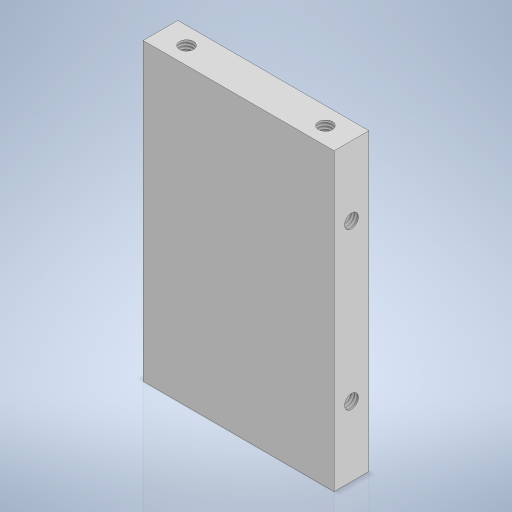
# Autodesk Inventor part: 1013
Saved by Autodesk Inventor 2024 (Build 280153000, 153)
## iProperties
Created: 2024-07-12
Part Number: 1013
Material: Generisch
Document SubType Name: Modeling
Designer: ffogue
Density: 1 g/cm^3
Appearance: Vorgabe
Author: ffogue
Autodesk Inventor part; units mm, degrees
ref_plane "XZ Plane" through (0, 0, 0) normal (0, 1, 0) x (-1, 0, 0)
sketch "Skizze1" plane through (0, 0, 0) normal (0, 1, 0) x (-1, 0, 0)
  line L0 (0, 0) -> (44, 0)
  line L1 (44, 0) -> (44, -68)
  line L2 (44, -68) -> (0, -68)
  line L3 (0, -68) -> (0, 0)
  dimension "d0" = 44
  dimension "d1" = 68
  constraints: 8 end point, 2 parallel, 1 horizontal, 1 perpendicular
  measures "d0" distance between parallel lines of L3 L1
  measures "d1" distance between parallel lines of L2 L0
extrude "Extrusion1" add sketch "Skizze1" along normal blind 8
sketch "Skizze2" plane through (-44, 0, 0) normal (0, 0, 1) x (1, 0, 0)
  line L0 (44, 0) -> (44, 8) projected
  point P0 (38, 4)
  point P1 (6, 4)
  point P2 (44, 4)
  dimension "d4" = 32
  dimension "d5" = 6
  constraints: 2 horizontal alignment, 1 midpoint
  measures "d4" distance of point (38, 4) point (6, 4)
  measures "d5" distance from line of L0 point (38, 4)
hole "Bohrung1" at (-6, 4, 0) at (-38, 4, 0) direction (0, 0, -1) diameter 3.242 depth 10 thread size "M4x0.7" class "6H" standard "ISO Metric profile"
ref_plane "Arbeitsebene1" through (0, 0, -34) normal (0, 0, 1) x (1, 0, 0)
mirror "Spiegeln1" about plane through (0, 0, -34) normal (0, 0, 1) of "Bohrung1"
sketch "Skizze3" plane through (-44, 0, -68) normal (-1, 0, 0) x (0, 0, 1)
  line L0 (68, 0) -> (68, 8) projected
  point P0 (52, 4)
  point P1 (16, 4)
  point P2 (68, 4)
  dimension "d21" = 16
  dimension "d22" = 36
  constraints: 2 horizontal alignment, 1 midpoint
  measures "d21" distance from line of point (52, 4) L0
  measures "d22" distance of point (16, 4) point (52, 4)
hole "Bohrung2" at (-44, 4, -16) at (-44, 4, -52) direction (1, 0, 0) diameter 3.242 depth 10 thread size "M4x0.7" class "6H" standard "ISO Metric profile"
ref_plane "Arbeitsebene2" through (-22, 0, 0) normal (1, 0, 0) x (0, 1, 0)
mirror "Spiegeln2" about plane through (-22, 0, 0) normal (1, 0, 0) of "Bohrung2"
